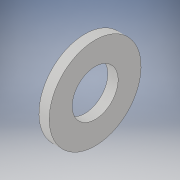
# Autodesk Inventor part: #10 Washer
Saved by Autodesk Inventor 2018 (Build 220112000, 112)
## iProperties
Created: 2019-01-23
Part Number: #10 Washer
Material: Generic
Document SubType Name: Modeling
Designer: s-2513398
Density: 1 g/cm^3
Appearance: Default
Author: s-2513398
Autodesk Inventor part; units mm, degrees
ref_plane "YZ Plane" through (0, 0, 0) normal (1, 0, 0) x (0, 1, 0)
ref_plane "XZ Plane" through (0, 0, 0) normal (0, 1, 0) x (-1, 0, 0)
ref_plane "XY Plane" through (0, 0, 0) normal (0, 0, 1) x (1, 0, 0)
sketch "Sketch1" plane through (0, 0, 0) normal (1, 0, 0) x (0, 1, 0)
  circle A0 centre (5.4452, 3.2344) radius 5.5563
  circle A1 centre (5.4452, 3.2344) radius 2.7781
  point P0 (0, 0)
  dimension "d0" = 11.1125
  dimension "d1" = 5.5563
  constraints: 2 centre point, 1 coincident
  measures "d0" diameter of A0
  measures "d1" diameter of A1
extrude "Extrusion1" add sketch "Sketch1" along normal blind 1.2446
body "Solid1"
